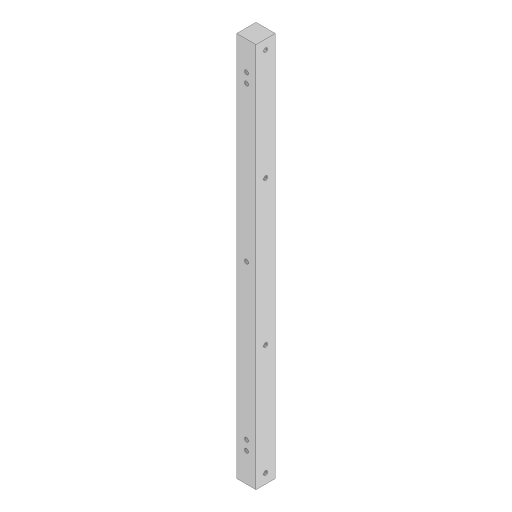
# Autodesk Inventor part: aluminium_stafmateriaal
Saved by Autodesk Inventor 2023 (Build 270158000, 158)
## iProperties
Created: 2022-09-12
Part Number: aluminium_stafmateriaal
Material: Aluminum 6061
Document SubType Name: Modeling
Designer: VoorL
Density: 2.7 g/cm^3
Appearance: Aluminum - Polished
Author: VoorL
Autodesk Inventor part; units mm, degrees
ref_plane "YZ Plane" through (0, 0, 0) normal (1, 0, 0) x (0, 1, 0)
ref_plane "XZ Plane" through (0, 0, 0) normal (0, 1, 0) x (-1, 0, 0)
ref_plane "XY Plane" through (0, 0, 0) normal (0, 0, 1) x (1, 0, 0)
sketch "Sketch1" plane through (0, 0, 0) normal (0, 1, 0) x (-1, 0, 0)
  line L0 (-10, 10) -> (10, 10)
  line L1 (10, 10) -> (10, -10)
  line L2 (10, -10) -> (-10, -10)
  line L3 (-10, -10) -> (-10, 10)
  line L4 (-10, 10) -> (10, -10) construction
  line L5 (10, 10) -> (-10, -10) construction
  point P0 (0, 0)
  dimension "d0" = 20
  dimension "d1" = 20
  constraints: 12 end point, 2 midpoint, 2 parallel, 1 horizontal, 1 perpendicular
  measures "d0" distance of L1.end L2.end
  measures "d1" distance of L0.end L1.end
extrude "Extrusion1" add sketch "Sketch1" along normal blind 400
sketch "Sketch2" plane through (10, 0, 10) normal (1, 0, 0) x (0, 0, -1)
  line L0 (10, 0) -> (10, 10)
  line L1 (10, 10) -> (10, 125)
  line L2 (10, 125) -> (10, 275)
  line L3 (10, 275) -> (10, 390)
  dimension "d4" = 10
  dimension "d5" = 115
  dimension "d6" = 150
  dimension "d7" = 180
  dimension "d8" = 115
  dimension "d9" = 180
  constraints: 8 end point, 2 collinear, 1 point on line, 1 vertical
  measures "d4" distance of L0.start L0.end
  measures "d5" distance of L0.end L1.end
  measures "d6" distance of L1.end L2.end
  measures "d7" angle of L2 L1
  measures "d8" distance of L2.end L3.end
  measures "d9" angle of L3 L2
hole "Hole1" at (10, 10, 0) at (10, 125, 0) at (10, 275, 0) at (10, 390, 0) direction (-1, 0, 0) diameter 3.242 end through all thread size "M4x0.7" class "6H" standard "ANSI Metric M Profile"
sketch "Sketch3" plane through (-10, 0, 10) normal (0, 0, 1) x (1, 0, 0)
  line L0 (10, 0) -> (10, 30)
  line L1 (10, 0) -> (40, 0) construction
  line L2 (10, 30) -> (10, 370)
  dimension "d17" = 30
  dimension "d18" = 90
  dimension "d19" = 340
  dimension "d20" = 180
  constraints: 6 end point, 1 collinear, 1 horizontal, 1 perpendicular, 1 vertical
  measures "d17" distance of L0.start L0.end
  measures "d18" angle of L1 L0
  measures "d19" distance of L0.end L2.end
  measures "d20" angle of L2 L0
hole "Hole2" at (0, 30, 10) at (0, 370, 10) direction (0, 0, -1) diameter 3.242 depth 47.25 tip angle 118 thread size "M4x0.7" class "6H" standard "ANSI Metric M Profile"
sketch "Sketch4" plane through (-10, 0, 10) normal (0, 0, 1) x (1, 0, 0)
  circle A0 centre (10, 30) radius 1.621 projected
  line L0 (10, 30) -> (10, 40)
  circle A1 centre (10, 370) radius 1.621 projected
  line L1 (10, 370) -> (10, 360)
  point P0 (10, 0)
  dimension "d37" = 10
  dimension "d38" = 10
  constraints: 4 end point, 2 vertical
  measures "d37" distance of L1.start L1.end
  measures "d38" distance of L0.start L0.end
hole "Hole3" at (0, 40, 10) at (0, 360, 10) direction (0, 0, -1) diameter 3.242 depth 51.25 tip angle 118 thread size "M4x0.7" class "6H" standard "ANSI Metric M Profile"
sketch "Sketch5" plane through (-10, 0, 10) normal (0, 0, 1) x (1, 0, 0)
  line L0 (20, 400) -> (0, 400) projected
  line L1 (10, 400) -> (10, 0)
  circle A0 centre (10, 200) radius 43.7231
  constraints: 2 end point, 2 midpoint, 1 centre point, 1 vertical
hole "Hole4" at (0, 200, 10) direction (0, 0, -1) diameter 3.242 depth 57.3 tip angle 118 thread size "M4x0.7" class "6H" standard "ANSI Metric M Profile"
chamfer "Chamfer1" distance 0.5 angle 45 18 edges at (10, 390, 1.621) (10, 275, 1.621) (10, 125, 1.621) (10, 10, 1.621) (0, 371.621, 10) (0, 31.621, 10) (0, 361.621, 10) (0, 41.621, 10) (0, 201.621, 10) (0, 201.621, -10) (0, 361.621, -10) (0, 41.621, -10) (0, 371.621, -10) (0, 31.621, -10) (-10, 390, 1.621) (-10, 275, 1.621) (-10, 125, 1.621) (-10, 10, 1.621)
body "Solid1"
